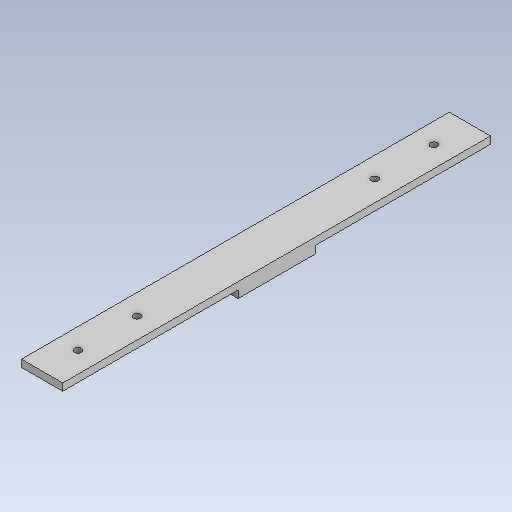
# Autodesk Inventor part: battery_support
Saved by Autodesk Inventor 2021 (Build 250183000, 183)
## iProperties
Created: 2021-03-02
Part Number: battery_support
Material: Generic
Document SubType Name: Modeling
Designer: Mateusz
Density: 1 g/cm^3
Appearance: Default
Author: Mateusz
Autodesk Inventor part; units mm, degrees
ref_plane "YZ Plane" through (0, 0, 0) normal (1, 0, 0) x (0, 1, 0)
ref_plane "XZ Plane" through (0, 0, 0) normal (0, 1, 0) x (-1, 0, 0)
ref_plane "XY Plane" through (0, 0, 0) normal (0, 0, 1) x (1, 0, 0)
sketch "Sketch1" plane through (0, 0, 0) normal (0, 1, 0) x (-1, 0, 0)
  line L0 (23, 0) -> (0, 0)
  line L1 (0, 0) -> (0, -238.782)
  line L2 (0, -238.782) -> (23, -238.782)
  line L3 (23, -238.782) -> (23, 0)
  dimension "d2" = 238.782
  constraints: 8 end point, 2 perpendicular, 1 vertical
  measures "d2" distance of L0.end L1.end
extrude "Extrusion1" add sketch "Sketch1" along normal blind 4
sketch "Sketch3" plane through (0, 0, 0) normal (0, -1, 0) x (1, 0, 0)
  line L0 (0, 0) -> (0, -238.782) projected
  line L1 (0, -119.391) -> (0, -136.891)
  line L2 (0, -136.891) -> (0, -101.891)
  line L3 (0, -101.891) -> (-23, -101.891)
  line L4 (-23, -238.782) -> (-23, 0) projected
  line L5 (-23, -101.891) -> (-23, -136.891)
  line L6 (0, -136.891) -> (-23, -136.891)
  dimension "d5" = 17.5
  dimension "d6" = 35
  constraints: 10 end point, 4 point on line, 2 perpendicular, 1 midpoint
  measures "d5" distance of L1.start L1.end
  measures "d6" distance of L1.end L2.end
extrude "Extrusion2" add sketch "Sketch3" along normal blind 4.15
sketch "Sketch4" plane through (0, 0, 0) normal (0, -1, 0) x (1, 0, 0)
  circle A0 centre (-11.5, -185.782) radius 2 projected
  circle A1 centre (-11.5, -218.782) radius 2 projected
  circle A2 centre (-11.5, -20) radius 2 projected
  circle A3 centre (-11.5, -53) radius 2 projected
  point P0 (0, 0)
extrude "Extrusion3" cut sketch "Sketch4" against normal up to surface (4 mm away)
sketch "Sketch5" plane through (-23, 0, -101.891) normal (0, 0, 1) x (1, 0, 0)
  line L0 (0, 0) -> (23, 0) projected
  line L1 (0, 0) -> (0, -4.15) projected
  line L2 (23, -4.15) -> (0, -4.15) projected
  line L3 (23, 0) -> (23, -4.15) projected
  point P0 (23, 0)
extrude "Extrusion4" add sketch "Sketch5" along normal blind 4
sketch "Sketch6" plane through (0, 0, -136.891) normal (0, 0, -1) x (-1, 0, 0)
  line L0 (0, 0) -> (23, 0) projected
  line L1 (0, 0) -> (0, -4.15) projected
  line L2 (23, -4.15) -> (0, -4.15) projected
  line L3 (23, 0) -> (23, -4.15) projected
extrude "Extrusion5" add sketch "Sketch6" along normal blind 4
body "Solid1"
